Autodesk Inventor part; units mm, degrees
(part 2 of 4)
  line L125 (-9.1415, 0.6255) -> (-9.1721, 0.4922) construction
  line L126 (-9.1721, 0.4922) -> (-9.2026, 0.3592) construction
  line L127 (-9.2026, 0.3592) -> (-9.297, 0.2867) construction
  line L128 (-9.297, 0.2867) -> (-9.4268, 0.2624) construction
  line L129 (-9.4268, 0.2624) -> (-9.8787, 0.1776) construction
  line L130 (-9.8787, 0.1776) -> (-10.3313, 0.0968) construction
  line L131 (-10.3313, 0.0968) -> (-10.7828, 0.0101) construction
  line L132 (-10.7828, 0.0101) -> (-10.8726, -0.0072) construction
  line L133 (-10.8726, -0.0072) -> (-10.9599, -0.0407) construction
  line L134 (-10.9599, -0.0407) -> (-11.0464, -0.0719) construction
  line L135 (-11.0464, -0.0719) -> (-11.1372, -0.1048) construction
  line L136 (-11.1372, -0.1048) -> (-11.1793, -0.178) construction
  line L137 (-11.1793, -0.178) -> (-11.202, -0.269) construction
  line L138 (-11.202, -0.269) -> (-11.2438, -0.4368) construction
  line L139 (-11.2438, -0.4368) -> (-11.2023, -0.5985) construction
  line L140 (-11.2023, -0.5985) -> (-11.1712, -0.7605) construction
  line L141 (-11.1712, -0.7605) -> (-11.1015, -1.1234) construction
  line L142 (-11.1015, -1.1234) -> (-11.0295, -1.4858) construction
  line L143 (-11.0295, -1.4858) -> (-10.9532, -1.8473) construction
  line L144 (-10.9532, -1.8473) -> (-10.9457, -1.8828) construction
  line L145 (-10.9457, -1.8828) -> (-10.9084, -1.9273) construction
  line L146 (-10.9084, -1.9273) -> (-10.8748, -1.9396) construction
  line L147 (-10.8748, -1.9396) -> (-10.4566, -2.0916) construction
  line L148 (-10.4566, -2.0916) -> (-10.0419, -2.2568) construction
  line L149 (-10.0419, -2.2568) -> (-9.6157, -2.3822) construction
  line L150 (-9.6157, -2.3822) -> (-8.9721, -2.5716) construction
  line L151 (-8.9721, -2.5716) -> (-8.3199, -2.7319) construction
  line L152 (-8.3199, -2.7319) -> (-7.6717, -2.9059) construction
  line L153 (-7.6717, -2.9059) -> (-7.5951, -2.9264) construction
  line L154 (-7.5951, -2.9264) -> (-7.5555, -2.8808) construction
  line L155 (-7.5555, -2.8808) -> (-7.5235, -2.8285) construction
  line L156 (-7.5235, -2.8285) -> (-7.4397, -2.692) construction
  line L157 (-7.4397, -2.692) -> (-7.4153, -2.5388) construction
  line L158 (-7.4153, -2.5388) -> (-7.442, -2.3849) construction
  line L159 (-7.442, -2.3849) -> (-7.5081, -2.0041) construction
  line L160 (-7.5081, -2.0041) -> (-7.582, -1.6246) construction
  line L161 (-7.582, -1.6246) -> (-7.6571, -1.2454) construction
  line L162 (-7.6571, -1.2454) -> (-7.746, -0.7971) construction
  line L163 (-7.746, -0.7971) -> (-7.8402, -0.3498) construction
  line L164 (-7.8402, -0.3498) -> (-7.9309, 0.0982) construction
  line L165 (-7.9309, 0.0982) -> (-7.9807, 0.3436) construction
  line L166 (-7.9807, 0.3436) -> (-8.0916, 0.4464) construction
  line L167 (-8.0916, 0.4464) -> (-8.3387, 0.4678) construction
  line L168 (-8.3387, 0.4678) -> (-8.4163, 0.4745) construction
  line L169 (-8.4163, 0.4745) -> (-8.4944, 0.4741) construction
  line L170 (-8.4944, 0.4741) -> (-8.5722, 0.4792) construction
  line L171 (-8.5722, 0.4792) -> (-8.6303, 0.483) construction
  line L172 (-8.6303, 0.483) -> (-8.6898, 0.4839) construction
  line L173 (-8.6898, 0.4839) -> (-8.7459, 0.4976) construction
  line L174 (-8.7459, 0.4976) -> (-8.9235, 0.5409) construction
  line L175 (-8.9235, 0.5409) -> (-8.992, 0.7175) construction
  line L176 (-8.992, 0.7175) -> (-8.8985, 0.8745) construction
  line L177 (-8.8985, 0.8745) -> (-8.7942, 1.0494) construction
  line L178 (-8.7942, 1.0494) -> (-8.6225, 1.1165) construction
  line L179 (-8.6225, 1.1165) -> (-8.4386, 1.1526) construction
  line L180 (-8.4386, 1.1526) -> (-8.2405, 1.1914) construction
  line L181 (-8.2405, 1.1914) -> (-8.0393, 1.2145) construction
  line L182 (-8.0393, 1.2145) -> (-7.8391, 1.2422) construction
  line L183 (-7.8391, 1.2422) -> (-7.4652, 1.294) construction
  line L184 (-7.4652, 1.294) -> (-7.0916, 1.348) construction
  line L185 (-7.0916, 1.348) -> (-6.7169, 1.3925) construction
  line L186 (-6.7169, 1.3925) -> (-6.6023, 1.4061) construction
  line L187 (-6.6023, 1.4061) -> (-6.4832, 1.401) construction
  line L188 (-6.4832, 1.401) -> (-6.3682, 1.3875) construction
  line L189 (-6.3682, 1.3875) -> (-6.2267, 1.3709) construction
  line L190 (-6.2267, 1.3709) -> (-6.1216, 1.2721) construction
  line L191 (-6.1216, 1.2721) -> (-6.1023, 1.1616) construction
  line L192 (-6.1023, 1.1616) -> (-6.0806, 1.0381) construction
  line L193 (-6.0806, 1.0381) -> (-6.1476, 0.8994) construction
  line L194 (-6.1476, 0.8994) -> (-6.2789, 0.8383) construction
  line L195 (-6.2789, 0.8383) -> (-6.3816, 0.7906) construction
  line L196 (-6.3816, 0.7906) -> (-6.4934, 0.761) construction
  line L197 (-6.4934, 0.761) -> (-6.6033, 0.7308) construction
  line L198 (-6.6033, 0.7308) -> (-6.8238, 0.6701) construction
  line L199 (-6.8238, 0.6701) -> (-6.9226, 0.5484) construction
  line L200 (-6.9226, 0.5484) -> (-6.8975, 0.3204) construction
  line L201 (-6.8975, 0.3204) -> (-6.8633, 0.0086) construction
  line L202 (-6.8633, 0.0086) -> (-6.8208, -0.3026) construction
  line L203 (-6.8208, -0.3026) -> (-6.7684, -0.6118) construction
  line L204 (-6.7684, -0.6118) -> (-6.6783, -1.144) construction
  line L205 (-6.6783, -1.144) -> (-6.5786, -1.6746) construction
  line L206 (-6.5786, -1.6746) -> (-6.481, -2.2055) construction
  line L207 (-6.481, -2.2055) -> (-6.467, -2.2818) construction
  line L208 (-6.467, -2.2818) -> (-6.4462, -2.3575) construction
  line L209 (-6.4462, -2.3575) -> (-6.421, -2.4308) construction
  line L210 (-6.421, -2.4308) -> (-6.3423, -2.6595) construction
  line L211 (-6.3423, -2.6595) -> (-6.1706, -2.751) construction
  line L212 (-6.1706, -2.751) -> (-5.9336, -2.7011) construction
  line L213 (-5.9336, -2.7011) -> (-5.7911, -2.6711) construction
  line L214 (-5.7911, -2.6711) -> (-5.6477, -2.6422) construction
  line L215 (-5.6477, -2.6422) -> (-5.5032, -2.6256) construction
  line L216 (-5.5032, -2.6256) -> (-5.3654, -2.6098) construction
  line L217 (-5.3654, -2.6098) -> (-5.2355, -2.6427) construction
  line L218 (-5.2355, -2.6427) -> (-5.1342, -2.7463) construction
  line L219 (-5.1342, -2.7463) -> (-4.9562, -2.9286) construction
  line L220 (-4.9562, -2.9286) -> (-5.0397, -3.2467) construction
  line L221 (-5.0397, -3.2467) -> (-5.2961, -3.3506) construction
  line L222 (-5.2961, -3.3506) -> (-5.3877, -3.3877) construction
  line L223 (-5.3877, -3.3877) -> (-5.4863, -3.4076) construction
  line L224 (-5.4863, -3.4076) -> (-5.5964, -3.4396) construction
  line L225 (-5.5964, -3.4396) -> (-5.5666, -3.452) construction
  line L226 (-5.5666, -3.452) -> (-5.5456, -3.4636) construction
  line L227 (-5.5456, -3.4636) -> (-5.5231, -3.4696) construction
  line L228 (-5.5231, -3.4696) -> (-4.46, -3.7519) construction
  line L229 (-4.46, -3.7519) -> (-3.4059, -4.0644) construction
  line L230 (-3.4059, -4.0644) -> (-2.3654, -4.4212) construction
  line L231 (-2.3654, -4.4212) -> (-2.0639, -4.5246) construction
  line L232 (-2.0639, -4.5246) -> (-1.761, -4.6318) construction
  line L233 (-1.761, -4.6318) -> (-1.5003, -4.8214) construction
  line L234 (-1.5003, -4.8214) -> (-1.3917, -4.9004) construction
  line L235 (-1.3917, -4.9004) -> (-1.2877, -4.9957) construction
  line L236 (-1.2877, -4.9957) -> (-1.209, -5.1036) construction
  line L237 (-1.209, -5.1036) -> (-1.0533, -5.3173) construction
  line L238 (-1.0533, -5.3173) -> (-1.0838, -5.5776) construction
  line L239 (-1.0838, -5.5776) -> (-1.263, -5.7724) construction
  line L240 (-1.263, -5.7724) -> (-1.4413, -5.9664) construction
  line L241 (-1.4413, -5.9664) -> (-1.6684, -6.0667) construction
  line L242 (-1.6684, -6.0667) -> (-1.9231, -6.0989) construction
  line L243 (-1.9231, -6.0989) -> (-2.3941, -6.1586) construction
  line L244 (-2.3941, -6.1586) -> (-2.8652, -6.2281) construction
  line L245 (-2.8652, -6.2281) -> (-3.3385, -6.2567) construction
  line L246 (-3.3385, -6.2567) -> (-4.0167, -6.2976) construction
  line L247 (-4.0167, -6.2976) -> (-4.697, -6.3272) construction
  line L248 (-4.697, -6.3272) -> (-5.3762, -6.3227) construction
  line L249 (-5.3762, -6.3227) -> (-6.4798, -6.3154) construction
  line L250 (-6.4798, -6.3154) -> (-7.5831, -6.275) construction
  line L251 (-7.5831, -6.275) -> (-8.6866, -6.2514) construction
  line L252 (-8.6866, -6.2514) -> (-9.3078, -6.2382) construction
  line L253 (-9.3078, -6.2382) -> (-9.9297, -6.2097) construction
  line L254 (-9.9297, -6.2097) -> (-10.5503, -6.2255) construction
  line L255 (-10.5503, -6.2255) -> (-11.385, -6.2468) construction
  line L256 (-11.385, -6.2468) -> (-12.2071, -6.3678) construction
  line L257 (-12.2071, -6.3678) -> (-12.9983, -6.6549) construction
  line L258 (-12.9983, -6.6549) -> (-13.5047, -6.8387) construction
  line L259 (-13.5047, -6.8387) -> (-13.9638, -7.1106) construction
  line L260 (-13.9638, -7.1106) -> (-14.4209, -7.39) construction
  line L261 (-14.4209, -7.39) -> (-14.9749, -7.7284) construction
  line L262 (-14.9749, -7.7284) -> (-15.5263, -8.0734) construction
  line L263 (-15.5263, -8.0734) -> (-16.098, -8.38) construction
  line L264 (-16.098, -8.38) -> (-16.8167, -8.7655) construction
  line L265 (-16.8167, -8.7655) -> (-17.5898, -9.0139) construction
  line L266 (-17.5898, -9.0139) -> (-18.3874, -9.1846) construction
  line L267 (-18.3874, -9.1846) -> (-19.1584, -9.3496) construction
  line L268 (-19.1584, -9.3496) -> (-19.9377, -9.4137) construction
  line L269 (-19.9377, -9.4137) -> (-20.7253, -9.3901) construction
  line L270 (-20.7253, -9.3901) -> (-21.2696, -9.3737) construction
  line L271 (-21.2696, -9.3737) -> (-21.8068, -9.3051) construction
  line L272 (-21.8068, -9.3051) -> (-22.3409, -9.1993) construction
  line L273 (-22.3409, -9.1993) -> (-22.8994, -9.0886) construction
  line L274 (-22.8994, -9.0886) -> (-23.4408, -8.9244) construction
  line L275 (-23.4408, -8.9244) -> (-23.9614, -8.6965) construction
  line L276 (-23.9614, -8.6965) -> (-24.7827, -8.3369) construction
  line L277 (-24.7827, -8.3369) -> (-25.5451, -7.8792) construction
  line L278 (-25.5451, -7.8792) -> (-26.1979, -7.2599) construction
  line L279 (-26.1979, -7.2599) -> (-26.6165, -6.8628) construction
  line L280 (-26.6165, -6.8628) -> (-27.0112, -6.4405) construction
  line L281 (-27.0112, -6.4405) -> (-27.4171, -6.03) construction
  line L282 (-27.4171, -6.03) -> (-27.5073, -5.9388) construction
  line L283 (-27.5073, -5.9388) -> (-27.5995, -5.8496) construction
  line L284 (-27.5995, -5.8496) -> (-27.6907, -5.7595) construction
  line L285 (-27.6907, -5.7595) -> (-27.6972, -5.7631) construction
  line L286 (-27.6972, -5.7631) -> (-27.7038, -5.7666) construction
  line L287 (-27.7038, -5.7666) -> (-27.7103, -5.7702) construction
  line L288 (-27.7103, -5.7702) -> (-27.7045, -5.7909) construction
  line L289 (-27.7045, -5.7909) -> (-27.6981, -5.8114) construction
  line L290 (-27.6981, -5.8114) -> (-27.6931, -5.8323) construction
  line L291 (-27.6931, -5.8323) -> (-27.6517, -6.0067) construction
  line L292 (-27.6517, -6.0067) -> (-27.597, -6.1793) construction
  line L293 (-27.597, -6.1793) -> (-27.5727, -6.356) construction
  line L294 (-27.5727, -6.356) -> (-27.5432, -6.5712) construction
  line L295 (-27.5432, -6.5712) -> (-27.7159, -6.7223) construction
  line L296 (-27.7159, -6.7223) -> (-27.9327, -6.695) construction
  line L297 (-27.9327, -6.695) -> (-28.1066, -6.6731) construction
  line L298 (-28.1066, -6.6731) -> (-28.2563, -6.5942) construction
  line L299 (-28.2563, -6.5942) -> (-28.4029, -6.5055) construction
  line L300 (-28.4029, -6.5055) -> (-28.723, -6.312) construction
  line L301 (-28.723, -6.312) -> (-28.988, -6.0549) construction
  line L302 (-28.988, -6.0549) -> (-29.2411, -5.7836) construction
  line L303 (-29.2411, -5.7836) -> (-29.3886, -5.6255) construction
  line L304 (-29.3886, -5.6255) -> (-29.5283, -5.4582) construction
  line L305 (-29.5283, -5.4582) -> (-29.6891, -5.3148) construction
  line L306 (-29.6891, -5.3148) -> (-29.8892, -5.1361) construction
  line L307 (-29.8892, -5.1361) -> (-30.1284, -5.0394) construction
  line L308 (-30.1284, -5.0394) -> (-30.4054, -5.0607) construction
  line L309 (-30.4054, -5.0607) -> (-30.6564, -5.08) construction
  line L310 (-30.6564, -5.08) -> (-30.8625, -5.1824) construction
  line L311 (-30.8625, -5.1824) -> (-31.0209, -5.3798) construction
  line L312 (-31.0209, -5.3798) -> (-31.16, -5.5532) construction
  line L313 (-31.16, -5.5532) -> (-31.2551, -5.7489) construction
  line L314 (-31.2551, -5.7489) -> (-31.3218, -5.9595) construction
  line L315 (-31.3218, -5.9595) -> (-31.4388, -6.3288) construction
  line L316 (-31.4388, -6.3288) -> (-31.6164, -6.6694) construction
  line L317 (-31.6164, -6.6694) -> (-31.8243, -6.9939) construction
  line L318 (-31.8243, -6.9939) -> (-31.9164, -7.1375) construction
  line L319 (-31.9164, -7.1375) -> (-32.0288, -7.2696) construction
  line L320 (-32.0288, -7.2696) -> (-32.1781, -7.3575) construction
  line L321 (-32.1781, -7.3575) -> (-32.2423, -7.3953) construction
  line L322 (-32.2423, -7.3953) -> (-32.3224, -7.4185) construction
  line L323 (-32.3224, -7.4185) -> (-32.397, -7.4237) construction
  line L324 (-32.397, -7.4237) -> (-32.5113, -7.4317) construction
  line L325 (-32.5113, -7.4317) -> (-32.5926, -7.3729) construction
  line L326 (-32.5926, -7.3729) -> (-32.6412, -7.2633) construction
  line L327 (-32.6412, -7.2633) -> (-32.7533, -7.0109) construction
  line L328 (-32.7533, -7.0109) -> (-32.7522, -6.7457) construction
  line L329 (-32.7522, -6.7457) -> (-32.7292, -6.4807) construction
  line L330 (-32.7292, -6.4807) -> (-32.6561, -5.6383) construction
  line L331 (-32.6561, -5.6383) -> (-32.4383, -4.8295) construction
  line L332 (-32.4383, -4.8295) -> (-32.1464, -4.0389) construction
  line L333 (-32.1464, -4.0389) -> (-32.0867, -3.877) construction
  line L334 (-32.0867, -3.877) -> (-32.0244, -3.7159) construction
  line L335 (-32.0244, -3.7159) -> (-31.9579, -3.5566) construction
  line L336 (-31.9579, -3.5566) -> (-31.9347, -3.5009) construction
  line L337 (-31.9347, -3.5009) -> (-31.9455, -3.479) construction
  line L338 (-31.9455, -3.479) -> (-32.002, -3.4635) construction
  line L339 (-32.002, -3.4635) -> (-32.5597, -3.31) construction
  line L340 (-32.5597, -3.31) -> (-33.1132, -3.1393) construction
  line L341 (-33.1132, -3.1393) -> (-33.6753, -3.004) construction
  line L342 (-33.6753, -3.004) -> (-34.5429, -2.7951) construction
  line L343 (-34.5429, -2.7951) -> (-35.4166, -2.6112) construction
  line L344 (-35.4166, -2.6112) -> (-36.2872, -2.4147) construction
  line L345 (-36.2872, -2.4147) -> (-36.9812, -2.2582) construction
  line L346 (-36.9812, -2.2582) -> (-37.6646, -2.0653) construction
  line L347 (-37.6646, -2.0653) -> (-38.3233, -1.7938) construction
  line L348 (-38.3233, -1.7938) -> (-38.6564, -1.6565) construction
  line L349 (-38.6564, -1.6565) -> (-38.9816, -1.5016) construction
  line L350 (-38.9816, -1.5016) -> (-39.2782, -1.2935) construction
  line L351 (-39.2782, -1.2935) -> (-39.3873, -1.2169) construction
  line L352 (-39.3873, -1.2169) -> (-39.48, -1.1241) construction
  line L353 (-39.48, -1.1241) -> (-39.5354, -1.0006) construction
  line L354 (-39.5354, -1.0006) -> (-39.6222, -0.8072) construction
  line L355 (-39.6222, -0.8072) -> (-39.6072, -0.6192) construction
  line L356 (-39.6072, -0.6192) -> (-39.4623, -0.4639) construction
  line L357 (-39.4623, -0.4639) -> (-39.3816, -0.3774) construction
  line L358 (-39.3816, -0.3774) -> (-39.2771, -0.3041) construction
  line L359 (-39.2771, -0.3041) -> (-39.17, -0.2526) construction
  line L360 (-39.17, -0.2526) -> (-38.7966, -0.0731) construction
  line L361 (-38.7966, -0.0731) -> (-38.3904, -0.0146) construction
  line L362 (-38.3904, -0.0146) -> (-37.9851, 0.0411) construction
  line L363 (-37.9851, 0.0411) -> (-37.8502, 0.0596) construction
  line L364 (-37.8502, 0.0596) -> (-37.7138, 0.0677) construction
  line L365 (-37.7138, 0.0677) -> (-37.5779, 0.079) construction
  line L366 (-37.5779, 0.079) -> (-37.5311, 0.0828) construction
  line L367 (-37.5311, 0.0828) -> (-37.5181, 0.0974) construction
  line L368 (-37.5181, 0.0974) -> (-37.5278, 0.1486) construction
  line L369 (-37.5278, 0.1486) -> (-37.6076, 0.5737) construction
  line L370 (-37.6076, 0.5737) -> (-37.6983, 0.9976) construction
  line L371 (-37.6983, 0.9976) -> (-37.7568, 1.4258) construction
  line L372 (-37.7568, 1.4258) -> (-37.8162, 1.8607) construction
  line L373 (-37.8162, 1.8607) -> (-37.8234, 2.3001) construction
  line L374 (-37.8234, 2.3001) -> (-37.755, 2.737) construction
  line L375 (-37.755, 2.737) -> (-37.7344, 2.8688) construction
  line L376 (-37.7344, 2.8688) -> (-37.6587, 2.9608) construction
  line L377 (-37.6587, 2.9608) -> (-37.529, 2.9842) construction
  line L378 (-37.529, 2.9842) -> (-37.2061, 3.0425) construction
  line L379 (-37.2061, 3.0425) -> (-36.8828, 3.1064) construction
  line L380 (-36.8828, 3.1064) -> (-36.5568, 3.1378) construction
  line L381 (-36.5568, 3.1378) -> (-36.2765, 3.1648) construction
  line L382 (-36.2765, 3.1648) -> (-35.9921, 3.1533) construction
  line L383 (-35.9921, 3.1533) -> (-35.7096, 3.1523) construction
  line L384 (-35.7096, 3.1523) -> (-35.5311, 3.1516) construction
  line L385 (-35.5311, 3.1516) -> (-35.3544, 3.13) construction
  line L386 (-35.3544, 3.13) -> (-35.1948, 3.0392) construction
  line L387 (-35.1948, 3.0392) -> (-35.0805, 2.9741) construction
  line L388 (-35.0805, 2.9741) -> (-35.003, 2.8762) construction
  line L389 (-35.003, 2.8762) -> (-34.9516, 2.7566) construction
  line L390 (-34.9516, 2.7566) -> (-34.862, 2.5478) construction
  line L391 (-34.862, 2.5478) -> (-34.8252, 2.3278) construction
  line L392 (-34.8252, 2.3278) -> (-34.8157, 2.1027) construction
  line L393 (-34.8157, 2.1027) -> (-34.8121, 2.0169) construction
  line L394 (-34.8121, 2.0169) -> (-34.8151, 1.9308) construction
  line L395 (-34.8151, 1.9308) -> (-34.8151, 1.8449) construction
  line L396 (-34.8151, 1.8449) -> (-34.807, 1.8426) construction
  line L397 (-34.807, 1.8426) -> (-34.7989, 1.8403) construction
  line L398 (-34.7989, 1.8403) -> (-34.7908, 1.838) construction
  spline S1 degree 3 poles (-10.8046, -2.6746) (-10.8049, -2.6785) (-10.8072, -2.6879) (-10.8063, -2.6971) (-10.7803, -2.9734) (-10.75, -3.2493) (-10.7292, -3.526) (-10.7136, -3.7324) (-10.7319, -3.9357) (-10.8435, -4.1189) (-10.9866, -4.3539) (-11.2778, -4.4375) (-11.5015, -4.3033) (-11.6301, -4.2262) (-11.6996, -4.0978) (-11.7608, -3.9671) (-12.0323, -3.3866) (-12.1854, -2.772) (-12.271, -2.1401) (-12.2917, -1.9874) (-12.3401, -1.8815) (-12.4777, -1.7932) (-12.9915, -1.4638) (-13.4224, -1.0367) (-13.8361, -0.5922) (-13.8769, -0.5484) (-13.9189, -0.5326) (-13.9761, -0.5314) (-14.1048, -0.5288) (-14.2353, -0.5324) (-14.3617, -0.512) (-14.5586, -0.4803) (-14.6622, -0.2857) (-14.5841, -0.1023) (-14.5536, -0.0307) (-14.4987, 0.0306) (-14.4527, 0.0999) (-14.4997, 0.1558) (-14.5529, 0.2189) (-14.6061, 0.282) (-15.0566, 0.8164) (-15.5463, 1.3081) (-16.128, 1.7028) (-16.9784, 2.2798) (-17.9224, 2.6173) (-18.9269, 2.7951) (-19.2333, 2.8493) (-19.5445, 2.8822) (-19.8549, 2.906) (-20.3614, 2.9449) (-20.8673, 2.9238) (-21.3726, 2.8668) (-21.9816, 2.7981) (-22.5798, 2.6806) (-23.1623, 2.4911) (-23.7885, 2.2873) (-24.3706, 1.9875) (-24.9124, 1.618) (-25.3363, 1.3289) (-25.7398, 1.0097) (-26.1481, 0.6983) (-26.5739, 0.3736) (-27.0196, 0.0859) (-27.5287, -0.0923) (-28.2067, -0.3296) (-28.9059, -0.464) (-29.6225, -0.4881) (-30.1801, -0.5069) (-30.7387, -0.4944) (-31.2969, -0.499) (-31.3887, -0.4997) (-31.4802, -0.5174) (-31.5721, -0.5251) (-31.603, -0.5277) (-31.6347, -0.5254) (-31.6656, -0.5218) (-31.7232, -0.5152) (-31.7805, -0.4991) (-31.8379, -0.4988) (-32.5935, -0.4951) (-33.3492, -0.493) (-34.1048, -0.4917) (-34.4607, -0.4912) (-34.8166, -0.4966) (-35.1725, -0.4937) (-35.9986, -0.487) (-36.8248, -0.4755) (-37.6486, -0.5569) (-38.0343, -0.595) (-38.4189, -0.6404) (-38.7866, -0.773) (-38.8072, -0.7804) (-38.8243, -0.7973) (-38.8431, -0.8098) (-38.8262, -0.8253) (-38.8114, -0.8442) (-38.7922, -0.8558) (-38.4004, -1.092) (-37.9807, -1.2643) (-37.5477, -1.4089) (-36.9677, -1.6025) (-36.3767, -1.7518) (-35.7788, -1.8784) (-35.2435, -1.9918) (-34.7108, -2.1178) (-34.1767, -2.2372) (-33.3526, -2.4216) (-32.5354, -2.6318) (-31.7305, -2.8878) (-31.6684, -2.9076) (-31.6405, -2.8931) (-31.6079, -2.841) (-31.5371, -2.7276) (-31.4631, -2.6156) (-31.3819, -2.5095) (-31.2437, -2.3292) (-31.063, -2.2407) (-30.8323, -2.2878) (-30.6949, -2.3159) (-30.5688, -2.3726) (-30.4548, -2.4553) (-29.9506, -2.821) (-29.5224, -3.2668) (-29.1131, -3.7318) (-28.9127, -3.9595) (-28.7294, -4.1961) (-28.4587, -4.3589) (-28.1812, -4.5258) (-27.9327, -4.7411) (-27.6712, -4.9349) (-27.648, -4.9521) (-27.6226, -4.9665) (-27.5822, -4.9924) (-27.5822, -4.944) (-27.5788, -4.9155) (-27.5827, -4.888) (-27.6204, -4.6229) (-27.657, -4.3577) (-27.6982, -4.0931) (-27.7858, -3.5307) (-27.8782, -2.969) (-27.9632, -2.4061) (-27.9801, -2.2942) (-27.9893, -2.1758) (-27.9718, -2.0652) (-27.9482, -1.9157) (-27.8419, -1.823) (-27.6939, -1.7885) (-27.5471, -1.7543) (-27.4144, -1.7824) (-27.3043, -1.8935) (-27.1869, -2.012) (-27.1473, -2.1672) (-27.1107, -2.3201) (-27.0474, -2.5847) (-26.9969, -2.8525) (-26.9392, -3.1186) (-26.8342, -3.6032) (-26.7294, -4.0879) (-26.6212, -4.5718) (-26.5735, -4.7852) (-26.5279, -4.9999) (-26.4629, -5.2082) (-26.4002, -5.4087) (-26.2543, -5.5304) (-26.0386, -5.5436) (-25.9177, -5.551) (-25.7949, -5.5483) (-25.6742, -5.5369) (-25.2463, -5.4967) (-24.831, -5.3903) (-24.4153, -5.287) (-24.1563, -5.2226) (-23.8956, -5.1707) (-23.6286, -5.2246) (-23.3911, -5.2725) (-23.195, -5.3854) (-23.0898, -5.6166) (-23.0018, -5.8099) (-23.0739, -5.9575) (-23.2803, -6.0122) (-24.101, -6.2296) (-24.9399, -6.3475) (-25.7786, -6.4663) (-25.87, -6.4792) (-25.9618, -6.4898) (-26.067, -6.5032) (-26.0389, -6.5371) (-26.0252, -6.5571) (-26.0081, -6.5737) (-25.7001, -6.8723) (-25.376, -7.1519) (-25.0219, -7.3949) (-24.3485, -7.8571) (-23.6204, -8.2039) (-22.8349, -8.4301) (-22.3167, -8.5793) (-21.79, -8.6915) (-21.2532, -8.7308) (-20.8485, -8.7604) (-20.44, -8.7586) (-20.034, -8.7452) (-19.4221, -8.7251) (-18.8161, -8.6439) (-18.22, -8.4998) (-17.4595, -8.3159) (-16.7344, -8.0394) (-16.0583, -7.6444) (-15.5733, -7.361) (-15.0953, -7.0654) (-14.6164, -6.7717) (-14.1471, -6.484) (-13.6663, -6.2202) (-13.1436, -6.0411) (-12.3452, -5.7674) (-11.5228, -5.6253) (-10.6798, -5.6092) (-9.8536, -5.5933) (-9.0279, -5.6198) (-8.2018, -5.6397) (-7.0916, -5.6664) (-5.982, -5.7441) (-4.8705, -5.7013) (-4.4493, -5.6851) (-4.0273, -5.6778) (-3.6074, -5.6442) (-3.0858, -5.6025) (-2.5658, -5.5397) (-2.0456, -5.4809) (-1.9626, -5.4714) (-1.8825, -5.4349) (-1.8011, -5.4109) (-1.8021, -5.4025) (-1.8031, -5.3941) (-1.8041, -5.3857) (-1.823, -5.3711) (-1.8401, -5.3529) (-1.861, -5.3426) (-2.0349, -5.2564) (-2.2024, -5.1502) (-2.385, -5.0902) (-3.152, -4.8384) (-3.9203, -4.5897) (-4.6943, -4.3607) (-5.3937, -4.1537) (-6.1028, -3.9797) (-6.8041, -3.7791) (-7.0583, -3.7064) (-7.3037, -3.6819) (-7.5647, -3.7375) (-7.7779, -3.7828) (-7.9978, -3.8063) (-8.2158, -3.8169) (-8.473, -3.8294) (-8.6584, -3.5989) (-8.5873, -3.3635) (-8.5839, -3.3524) (-8.5838, -3.3404) (-8.5835, -3.3387) (-9.3253, -3.1169) (-10.0622, -2.8966) (-10.8046, -2.6746) knots 0 0 0 0 1 1 1 2 2 2 3 3 3 4 4 4 5 5 5 6 6 6 7 7 7 8 8 8 9 9 9 10 10 10 11 11 11 12 12 12 13 13 13 14 14 14 15 15 15 16 16 16 17 17 17 18 18 18 19 19 19 20 20 20 21 21 21 22 22 22 23 23 23 24 24 24 25 25 25 26 26 26 27 27 27 28 28 28 29 29 29 30 30 30 31 31 31 32 32 32 33 33 33 34 34 34 35 35 35 36 36 36 37 37 37 38 38 38 39 39 39 40 40 40 41 41 41 42 42 42 43 43 43 44 44 44 45 45 45 46 46 46 47 47 47 48 48 48 49 49 49 50 50 50 51 51 51 52 52 52 53 53 53 54 54 54 55 55 55 56 56 56 57 57 57 58 58 58 59 59 59 60 60 60 61 61 61 62 62 62 63 63 63 64 64 64 65 65 65 66 66 66 67 67 67 68 68 68 69 69 69 70 70 70 71 71 71 72 72 72 73 73 73 74 74 74 75 75 75 76 76 76 77 77 77 78 78 78 79 79 79 80 80 80 81 81 81 82 82 82 83 83 83 84 84 84 85 85 85 86 86 86 87 87 87 87
  line L399 (-10.8046, -2.6746) -> (-10.8049, -2.6785) construction
  line L400 (-10.8049, -2.6785) -> (-10.8072, -2.6879) construction
  line L401 (-10.8072, -2.6879) -> (-10.8063, -2.6971) construction
  line L402 (-10.8063, -2.6971) -> (-10.7803, -2.9734) construction
  line L403 (-10.7803, -2.9734) -> (-10.75, -3.2493) construction
  line L404 (-10.75, -3.2493) -> (-10.7292, -3.526) construction
  line L405 (-10.7292, -3.526) -> (-10.7136, -3.7324) construction
  line L406 (-10.7136, -3.7324) -> (-10.7319, -3.9357) construction
  line L407 (-10.7319, -3.9357) -> (-10.8435, -4.1189) construction
  line L408 (-10.8435, -4.1189) -> (-10.9866, -4.3539) construction
  line L409 (-10.9866, -4.3539) -> (-11.2778, -4.4375) construction
  line L410 (-11.2778, -4.4375) -> (-11.5015, -4.3033) construction
  line L411 (-11.5015, -4.3033) -> (-11.6301, -4.2262) construction
  line L412 (-11.6301, -4.2262) -> (-11.6996, -4.0978) construction
  line L413 (-11.6996, -4.0978) -> (-11.7608, -3.9671) construction
  line L414 (-11.7608, -3.9671) -> (-12.0323, -3.3866) construction
  line L415 (-12.0323, -3.3866) -> (-12.1854, -2.772) construction
  line L416 (-12.1854, -2.772) -> (-12.271, -2.1401) construction
  line L417 (-12.271, -2.1401) -> (-12.2917, -1.9874) construction
  line L418 (-12.2917, -1.9874) -> (-12.3401, -1.8815) construction
  line L419 (-12.3401, -1.8815) -> (-12.4777, -1.7932) construction
  line L420 (-12.4777, -1.7932) -> (-12.9915, -1.4638) construction
  line L421 (-12.9915, -1.4638) -> (-13.4224, -1.0367) construction
  line L422 (-13.4224, -1.0367) -> (-13.8361, -0.5922) construction
  line L423 (-13.8361, -0.5922) -> (-13.8769, -0.5484) construction
  line L424 (-13.8769, -0.5484) -> (-13.9189, -0.5326) construction
  line L425 (-13.9189, -0.5326) -> (-13.9761, -0.5314) construction
  line L426 (-13.9761, -0.5314) -> (-14.1048, -0.5288) construction
  line L427 (-14.1048, -0.5288) -> (-14.2353, -0.5324) construction
  line L428 (-14.2353, -0.5324) -> (-14.3617, -0.512) construction
  line L429 (-14.3617, -0.512) -> (-14.5586, -0.4803) construction
  line L430 (-14.5586, -0.4803) -> (-14.6622, -0.2857) construction
  line L431 (-14.6622, -0.2857) -> (-14.5841, -0.1023) construction
  line L432 (-14.5841, -0.1023) -> (-14.5536, -0.0307) construction
  line L433 (-14.5536, -0.0307) -> (-14.4987, 0.0306) construction
  line L434 (-14.4987, 0.0306) -> (-14.4527, 0.0999) construction
  line L435 (-14.4527, 0.0999) -> (-14.4997, 0.1558) construction
  line L436 (-14.4997, 0.1558) -> (-14.5529, 0.2189) construction
  line L437 (-14.5529, 0.2189) -> (-14.6061, 0.282) construction
  line L438 (-14.6061, 0.282) -> (-15.0566, 0.8164) construction
  line L439 (-15.0566, 0.8164) -> (-15.5463, 1.3081) construction
  line L440 (-15.5463, 1.3081) -> (-16.128, 1.7028) construction
  line L441 (-16.128, 1.7028) -> (-16.9784, 2.2798) construction
  line L442 (-16.9784, 2.2798) -> (-17.9224, 2.6173) construction
  line L443 (-17.9224, 2.6173) -> (-18.9269, 2.7951) construction
  line L444 (-18.9269, 2.7951) -> (-19.2333, 2.8493) construction
  line L445 (-19.2333, 2.8493) -> (-19.5445, 2.8822) construction
  line L446 (-19.5445, 2.8822) -> (-19.8549, 2.906) construction
  line L447 (-19.8549, 2.906) -> (-20.3614, 2.9449) construction
  line L448 (-20.3614, 2.9449) -> (-20.8673, 2.9238) construction
  line L449 (-20.8673, 2.9238) -> (-21.3726, 2.8668) construction
  line L450 (-21.3726, 2.8668) -> (-21.9816, 2.7981) construction
  line L451 (-21.9816, 2.7981) -> (-22.5798, 2.6806) construction
  line L452 (-22.5798, 2.6806) -> (-23.1623, 2.4911) construction
  line L453 (-23.1623, 2.4911) -> (-23.7885, 2.2873) construction
  line L454 (-23.7885, 2.2873) -> (-24.3706, 1.9875) construction
  line L455 (-24.3706, 1.9875) -> (-24.9124, 1.618) construction
  line L456 (-24.9124, 1.618) -> (-25.3363, 1.3289) construction
  line L457 (-25.3363, 1.3289) -> (-25.7398, 1.0097) construction
  line L458 (-25.7398, 1.0097) -> (-26.1481, 0.6983) construction
  line L459 (-26.1481, 0.6983) -> (-26.5739, 0.3736) construction
  line L460 (-26.5739, 0.3736) -> (-27.0196, 0.0859) construction
  line L461 (-27.0196, 0.0859) -> (-27.5287, -0.0923) construction
  line L462 (-27.5287, -0.0923) -> (-28.2067, -0.3296) construction
  line L463 (-28.2067, -0.3296) -> (-28.9059, -0.464) construction
  line L464 (-28.9059, -0.464) -> (-29.6225, -0.4881) construction
  line L465 (-29.6225, -0.4881) -> (-30.1801, -0.5069) construction
  line L466 (-30.1801, -0.5069) -> (-30.7387, -0.4944) construction
  line L467 (-30.7387, -0.4944) -> (-31.2969, -0.499) construction
  line L468 (-31.2969, -0.499) -> (-31.3887, -0.4997) construction
  line L469 (-31.3887, -0.4997) -> (-31.4802, -0.5174) construction
  line L470 (-31.4802, -0.5174) -> (-31.5721, -0.5251) construction
  line L471 (-31.5721, -0.5251) -> (-31.603, -0.5277) construction
  line L472 (-31.603, -0.5277) -> (-31.6347, -0.5254) construction
  line L473 (-31.6347, -0.5254) -> (-31.6656, -0.5218) construction
  line L474 (-31.6656, -0.5218) -> (-31.7232, -0.5152) construction
  line L475 (-31.7232, -0.5152) -> (-31.7805, -0.4991) construction
  line L476 (-31.7805, -0.4991) -> (-31.8379, -0.4988) construction
  line L477 (-31.8379, -0.4988) -> (-32.5935, -0.4951) construction
  line L478 (-32.5935, -0.4951) -> (-33.3492, -0.493) construction
  line L479 (-33.3492, -0.493) -> (-34.1048, -0.4917) construction
  line L480 (-34.1048, -0.4917) -> (-34.4607, -0.4912) construction
  line L481 (-34.4607, -0.4912) -> (-34.8166, -0.4966) construction
  line L482 (-34.8166, -0.4966) -> (-35.1725, -0.4937) construction
  line L483 (-35.1725, -0.4937) -> (-35.9986, -0.487) construction
  line L484 (-35.9986, -0.487) -> (-36.8248, -0.4755) construction
  line L485 (-36.8248, -0.4755) -> (-37.6486, -0.5569) construction
  line L486 (-37.6486, -0.5569) -> (-38.0343, -0.595) construction
  line L487 (-38.0343, -0.595) -> (-38.4189, -0.6404) construction
  line L488 (-38.4189, -0.6404) -> (-38.7866, -0.773) construction
  line L489 (-38.7866, -0.773) -> (-38.8072, -0.7804) construction
  line L490 (-38.8072, -0.7804) -> (-38.8243, -0.7973) construction
  line L491 (-38.8243, -0.7973) -> (-38.8431, -0.8098) construction
  line L492 (-38.8431, -0.8098) -> (-38.8262, -0.8253) construction
  line L493 (-38.8262, -0.8253) -> (-38.8114, -0.8442) construction
  line L494 (-38.8114, -0.8442) -> (-38.7922, -0.8558) construction
  line L495 (-38.7922, -0.8558) -> (-38.4004, -1.092) construction
  line L496 (-38.4004, -1.092) -> (-37.9807, -1.2643) construction
  line L497 (-37.9807, -1.2643) -> (-37.5477, -1.4089) construction
  line L498 (-37.5477, -1.4089) -> (-36.9677, -1.6025) construction
  line L499 (-36.9677, -1.6025) -> (-36.3767, -1.7518) construction
  line L500 (-36.3767, -1.7518) -> (-35.7788, -1.8784) construction
  line L501 (-35.7788, -1.8784) -> (-35.2435, -1.9918) construction
  line L502 (-35.2435, -1.9918) -> (-34.7108, -2.1178) construction
  line L503 (-34.7108, -2.1178) -> (-34.1767, -2.2372) construction
  line L504 (-34.1767, -2.2372) -> (-33.3526, -2.4216) construction
  line L505 (-33.3526, -2.4216) -> (-32.5354, -2.6318) construction
  line L506 (-32.5354, -2.6318) -> (-31.7305, -2.8878) construction
  line L507 (-31.7305, -2.8878) -> (-31.6684, -2.9076) construction
  line L508 (-31.6684, -2.9076) -> (-31.6405, -2.8931) construction
  line L509 (-31.6405, -2.8931) -> (-31.6079, -2.841) construction
  line L510 (-31.6079, -2.841) -> (-31.5371, -2.7276) construction
  line L511 (-31.5371, -2.7276) -> (-31.4631, -2.6156) construction
  line L512 (-31.4631, -2.6156) -> (-31.3819, -2.5095) construction
  line L513 (-31.3819, -2.5095) -> (-31.2437, -2.3292) construction
  line L514 (-31.2437, -2.3292) -> (-31.063, -2.2407) construction
  line L515 (-31.063, -2.2407) -> (-30.8323, -2.2878) construction
  line L516 (-30.8323, -2.2878) -> (-30.6949, -2.3159) construction
  line L517 (-30.6949, -2.3159) -> (-30.5688, -2.3726) construction
  line L518 (-30.5688, -2.3726) -> (-30.4548, -2.4553) construction
  line L519 (-30.4548, -2.4553) -> (-29.9506, -2.821) construction
  line L520 (-29.9506, -2.821) -> (-29.5224, -3.2668) construction
  line L521 (-29.5224, -3.2668) -> (-29.1131, -3.7318) construction
  line L522 (-29.1131, -3.7318) -> (-28.9127, -3.9595) construction
  line L523 (-28.9127, -3.9595) -> (-28.7294, -4.1961) construction
  line L524 (-28.7294, -4.1961) -> (-28.4587, -4.3589) construction
  line L525 (-28.4587, -4.3589) -> (-28.1812, -4.5258) construction
  line L526 (-28.1812, -4.5258) -> (-27.9327, -4.7411) construction
  line L527 (-27.9327, -4.7411) -> (-27.6712, -4.9349) construction
  line L528 (-27.6712, -4.9349) -> (-27.648, -4.9521) construction
  line L529 (-27.648, -4.9521) -> (-27.6226, -4.9665) construction
  line L530 (-27.6226, -4.9665) -> (-27.5822, -4.9924) construction
  line L531 (-27.5822, -4.9924) -> (-27.5822, -4.944) construction
  line L532 (-27.5822, -4.944) -> (-27.5788, -4.9155) construction
  line L533 (-27.5788, -4.9155) -> (-27.5827, -4.888) construction
  line L534 (-27.5827, -4.888) -> (-27.6204, -4.6229) construction
  line L535 (-27.6204, -4.6229) -> (-27.657, -4.3577) construction
  line L536 (-27.657, -4.3577) -> (-27.6982, -4.0931) construction
  line L537 (-27.6982, -4.0931) -> (-27.7858, -3.5307) construction
  line L538 (-27.7858, -3.5307) -> (-27.8782, -2.969) construction
  line L539 (-27.8782, -2.969) -> (-27.9632, -2.4061) construction
  line L540 (-27.9632, -2.4061) -> (-27.9801, -2.2942) construction
  line L541 (-27.9801, -2.2942) -> (-27.9893, -2.1758) construction
  line L542 (-27.9893, -2.1758) -> (-27.9718, -2.0652) construction
  line L543 (-27.9718, -2.0652) -> (-27.9482, -1.9157) construction
  line L544 (-27.9482, -1.9157) -> (-27.8419, -1.823) construction
  line L545 (-27.8419, -1.823) -> (-27.6939, -1.7885) construction
  line L546 (-27.6939, -1.7885) -> (-27.5471, -1.7543) construction
  line L547 (-27.5471, -1.7543) -> (-27.4144, -1.7824) construction
  line L548 (-27.4144, -1.7824) -> (-27.3043, -1.8935) construction
  line L549 (-27.3043, -1.8935) -> (-27.1869, -2.012) construction
  line L550 (-27.1869, -2.012) -> (-27.1473, -2.1672) construction
  line L551 (-27.1473, -2.1672) -> (-27.1107, -2.3201) construction
  line L552 (-27.1107, -2.3201) -> (-27.0474, -2.5847) construction
  line L553 (-27.0474, -2.5847) -> (-26.9969, -2.8525) construction
  line L554 (-26.9969, -2.8525) -> (-26.9392, -3.1186) construction
  line L555 (-26.9392, -3.1186) -> (-26.8342, -3.6032) construction
  line L556 (-26.8342, -3.6032) -> (-26.7294, -4.0879) construction
  line L557 (-26.7294, -4.0879) -> (-26.6212, -4.5718) construction
  line L558 (-26.6212, -4.5718) -> (-26.5735, -4.7852) construction
  line L559 (-26.5735, -4.7852) -> (-26.5279, -4.9999) construction
  line L560 (-26.5279, -4.9999) -> (-26.4629, -5.2082) construction
  line L561 (-26.4629, -5.2082) -> (-26.4002, -5.4087) construction
  line L562 (-26.4002, -5.4087) -> (-26.2543, -5.5304) construction
  line L563 (-26.2543, -5.5304) -> (-26.0386, -5.5436) construction
  line L564 (-26.0386, -5.5436) -> (-25.9177, -5.551) construction
  line L565 (-25.9177, -5.551) -> (-25.7949, -5.5483) construction
  line L566 (-25.7949, -5.5483) -> (-25.6742, -5.5369) construction
  line L567 (-25.6742, -5.5369) -> (-25.2463, -5.4967) construction
  line L568 (-25.2463, -5.4967) -> (-24.831, -5.3903) construction
  line L569 (-24.831, -5.3903) -> (-24.4153, -5.287) construction
  line L570 (-24.4153, -5.287) -> (-24.1563, -5.2226) construction
  line L571 (-24.1563, -5.2226) -> (-23.8956, -5.1707) construction
  line L572 (-23.8956, -5.1707) -> (-23.6286, -5.2246) construction
  line L573 (-23.6286, -5.2246) -> (-23.3911, -5.2725) construction
  line L574 (-23.3911, -5.2725) -> (-23.195, -5.3854) construction
  line L575 (-23.195, -5.3854) -> (-23.0898, -5.6166) construction
  line L576 (-23.0898, -5.6166) -> (-23.0018, -5.8099) construction
  line L577 (-23.0018, -5.8099) -> (-23.0739, -5.9575) construction
  line L578 (-23.0739, -5.9575) -> (-23.2803, -6.0122) construction
  line L579 (-23.2803, -6.0122) -> (-24.101, -6.2296) construction
  line L580 (-24.101, -6.2296) -> (-24.9399, -6.3475) construction
  line L581 (-24.9399, -6.3475) -> (-25.7786, -6.4663) construction
  line L582 (-25.7786, -6.4663) -> (-25.87, -6.4792) construction
  line L583 (-25.87, -6.4792) -> (-25.9618, -6.4898) construction
  line L584 (-25.9618, -6.4898) -> (-26.067, -6.5032) construction
  line L585 (-26.067, -6.5032) -> (-26.0389, -6.5371) construction
  line L586 (-26.0389, -6.5371) -> (-26.0252, -6.5571) construction
  line L587 (-26.0252, -6.5571) -> (-26.0081, -6.5737) construction
  line L588 (-26.0081, -6.5737) -> (-25.7001, -6.8723) construction
  line L589 (-25.7001, -6.8723) -> (-25.376, -7.1519) construction
  line L590 (-25.376, -7.1519) -> (-25.0219, -7.3949) construction
  line L591 (-25.0219, -7.3949) -> (-24.3485, -7.8571) construction
  line L592 (-24.3485, -7.8571) -> (-23.6204, -8.2039) construction
  line L593 (-23.6204, -8.2039) -> (-22.8349, -8.4301) construction
  line L594 (-22.8349, -8.4301) -> (-22.3167, -8.5793) construction
  line L595 (-22.3167, -8.5793) -> (-21.79, -8.6915) construction
  line L596 (-21.79, -8.6915) -> (-21.2532, -8.7308) construction
  line L597 (-21.2532, -8.7308) -> (-20.8485, -8.7604) construction
  line L598 (-20.8485, -8.7604) -> (-20.44, -8.7586) construction
  line L599 (-20.44, -8.7586) -> (-20.034, -8.7452) construction
  line L600 (-20.034, -8.7452) -> (-19.4221, -8.7251) construction
  line L601 (-19.4221, -8.7251) -> (-18.8161, -8.6439) construction
  line L602 (-18.8161, -8.6439) -> (-18.22, -8.4998) construction
  line L603 (-18.22, -8.4998) -> (-17.4595, -8.3159) construction
  line L604 (-17.4595, -8.3159) -> (-16.7344, -8.0394) construction
  line L605 (-16.7344, -8.0394) -> (-16.0583, -7.6444) construction
  line L606 (-16.0583, -7.6444) -> (-15.5733, -7.361) construction
  line L607 (-15.5733, -7.361) -> (-15.0953, -7.0654) construction
  line L608 (-15.0953, -7.0654) -> (-14.6164, -6.7717) construction
  line L609 (-14.6164, -6.7717) -> (-14.1471, -6.484) construction
  line L610 (-14.1471, -6.484) -> (-13.6663, -6.2202) construction
  line L611 (-13.6663, -6.2202) -> (-13.1436, -6.0411) construction
  line L612 (-13.1436, -6.0411) -> (-12.3452, -5.7674) construction
  line L613 (-12.3452, -5.7674) -> (-11.5228, -5.6253) construction
  line L614 (-11.5228, -5.6253) -> (-10.6798, -5.6092) construction
  line L615 (-10.6798, -5.6092) -> (-9.8536, -5.5933) construction
  line L616 (-9.8536, -5.5933) -> (-9.0279, -5.6198) construction
  line L617 (-9.0279, -5.6198) -> (-8.2018, -5.6397) construction
  line L618 (-8.2018, -5.6397) -> (-7.0916, -5.6664) construction
  line L619 (-7.0916, -5.6664) -> (-5.982, -5.7441) construction
  line L620 (-5.982, -5.7441) -> (-4.8705, -5.7013) construction
  line L621 (-4.8705, -5.7013) -> (-4.4493, -5.6851) construction
  line L622 (-4.4493, -5.6851) -> (-4.0273, -5.6778) construction
  line L623 (-4.0273, -5.6778) -> (-3.6074, -5.6442) construction
  line L624 (-3.6074, -5.6442) -> (-3.0858, -5.6025) construction
  line L625 (-3.0858, -5.6025) -> (-2.5658, -5.5397) construction
  line L626 (-2.5658, -5.5397) -> (-2.0456, -5.4809) construction
  line L627 (-2.0456, -5.4809) -> (-1.9626, -5.4714) construction
  line L628 (-1.9626, -5.4714) -> (-1.8825, -5.4349) construction
  line L629 (-1.8825, -5.4349) -> (-1.8011, -5.4109) construction
  line L630 (-1.8011, -5.4109) -> (-1.8021, -5.4025) construction
  line L631 (-1.8021, -5.4025) -> (-1.8031, -5.3941) construction
  line L632 (-1.8031, -5.3941) -> (-1.8041, -5.3857) construction
  line L633 (-1.8041, -5.3857) -> (-1.823, -5.3711) construction
  line L634 (-1.823, -5.3711) -> (-1.8401, -5.3529) construction
  line L635 (-1.8401, -5.3529) -> (-1.861, -5.3426) construction
  line L636 (-1.861, -5.3426) -> (-2.0349, -5.2564) construction
  line L637 (-2.0349, -5.2564) -> (-2.2024, -5.1502) construction
  line L638 (-2.2024, -5.1502) -> (-2.385, -5.0902) construction
  line L639 (-2.385, -5.0902) -> (-3.152, -4.8384) construction
  line L640 (-3.152, -4.8384) -> (-3.9203, -4.5897) construction
  line L641 (-3.9203, -4.5897) -> (-4.6943, -4.3607) construction
  line L642 (-4.6943, -4.3607) -> (-5.3937, -4.1537) construction
  line L643 (-5.3937, -4.1537) -> (-6.1028, -3.9797) construction
  line L644 (-6.1028, -3.9797) -> (-6.8041, -3.7791) construction
  line L645 (-6.8041, -3.7791) -> (-7.0583, -3.7064) construction
  line L646 (-7.0583, -3.7064) -> (-7.3037, -3.6819) construction
  line L647 (-7.3037, -3.6819) -> (-7.5647, -3.7375) construction
  line L648 (-7.5647, -3.7375) -> (-7.7779, -3.7828) construction
  line L649 (-7.7779, -3.7828) -> (-7.9978, -3.8063) construction
  line L650 (-7.9978, -3.8063) -> (-8.2158, -3.8169) construction
  line L651 (-8.2158, -3.8169) -> (-8.473, -3.8294) construction
  line L652 (-8.473, -3.8294) -> (-8.6584, -3.5989) construction
  line L653 (-8.6584, -3.5989) -> (-8.5873, -3.3635) construction
  line L654 (-8.5873, -3.3635) -> (-8.5839, -3.3524) construction
  line L655 (-8.5839, -3.3524) -> (-8.5838, -3.3404) construction
  line L656 (-8.5838, -3.3404) -> (-8.5835, -3.3387) construction
  line L657 (-8.5835, -3.3387) -> (-9.3253, -3.1169) construction
  line L658 (-9.3253, -3.1169) -> (-10.0622, -2.8966) construction
  line L659 (-10.0622, -2.8966) -> (-10.8046, -2.6746) construction
  spline S2 degree 3 poles (-36.9183, 1.2424) (-36.9146, 1.2037) (-36.91, 1.1614) (-36.9065, 1.1191) (-36.8811, 0.8134) (-36.855, 0.5079) (-36.8315, 0.2021) (-36.8273, 0.1474) (-36.8096, 0.1264) (-36.7512, 0.1286) (-36.5712, 0.1357) (-36.3909, 0.139) (-36.2107, 0.1399) (-35.9136, 0.1414) (-35.6164, 0.138) (-35.3193, 0.1406) (-35.1758, 0.1419) (-35.1823, 0.1473) (-35.1557, 0.2864) (-35.0965, 0.5966) (-35.0299, 0.9055) (-34.9669, 1.215) (-34.9615, 1.2412) (-34.9598, 1.2682) (-34.9579, 1.283) (-35.0599, 1.235) (-35.1542, 1.1676) (-35.2581, 1.146) (-35.57, 1.0809) (-35.8877, 1.079) (-36.203, 1.1193) (-36.4382, 1.1494) (-36.6709, 1.199) (-36.9183, 1.2424) knots 0 0 0 0 1 1 1 2 2 2 3 3 3 4 4 4 5 5 5 6 6 6 7 7 7 8 8 8 9 9 9 10 10 10 11 11 11 11
  line L660 (-36.9183, 1.2424) -> (-36.9146, 1.2037) construction
  line L661 (-36.9146, 1.2037) -> (-36.91, 1.1614) construction
  line L662 (-36.91, 1.1614) -> (-36.9065, 1.1191) construction
  line L663 (-36.9065, 1.1191) -> (-36.8811, 0.8134) construction
  line L664 (-36.8811, 0.8134) -> (-36.855, 0.5079) construction
  line L665 (-36.855, 0.5079) -> (-36.8315, 0.2021) construction
  line L666 (-36.8315, 0.2021) -> (-36.8273, 0.1474) construction
  line L667 (-36.8273, 0.1474) -> (-36.8096, 0.1264) construction
  line L668 (-36.8096, 0.1264) -> (-36.7512, 0.1286) construction
  line L669 (-36.7512, 0.1286) -> (-36.5712, 0.1357) construction
  line L670 (-36.5712, 0.1357) -> (-36.3909, 0.139) construction
  line L671 (-36.3909, 0.139) -> (-36.2107, 0.1399) construction
  line L672 (-36.2107, 0.1399) -> (-35.9136, 0.1414) construction
  line L673 (-35.9136, 0.1414) -> (-35.6164, 0.138) construction
  line L674 (-35.6164, 0.138) -> (-35.3193, 0.1406) construction
  line L675 (-35.3193, 0.1406) -> (-35.1758, 0.1419) construction
  line L676 (-35.1758, 0.1419) -> (-35.1823, 0.1473) construction
  line L677 (-35.1823, 0.1473) -> (-35.1557, 0.2864) construction
  line L678 (-35.1557, 0.2864) -> (-35.0965, 0.5966) construction
  line L679 (-35.0965, 0.5966) -> (-35.0299, 0.9055) construction
  line L680 (-35.0299, 0.9055) -> (-34.9669, 1.215) construction
  line L681 (-34.9669, 1.215) -> (-34.9615, 1.2412) construction
  line L682 (-34.9615, 1.2412) -> (-34.9598, 1.2682) construction
  line L683 (-34.9598, 1.2682) -> (-34.9579, 1.283) construction
  line L684 (-34.9579, 1.283) -> (-35.0599, 1.235) construction
  line L685 (-35.0599, 1.235) -> (-35.1542, 1.1676) construction
  line L686 (-35.1542, 1.1676) -> (-35.2581, 1.146) construction
  line L687 (-35.2581, 1.146) -> (-35.57, 1.0809) construction
  line L688 (-35.57, 1.0809) -> (-35.8877, 1.079) construction
  line L689 (-35.8877, 1.079) -> (-36.203, 1.1193) construction
  line L690 (-36.203, 1.1193) -> (-36.4382, 1.1494) construction
  line L691 (-36.4382, 1.1494) -> (-36.6709, 1.199) construction
  line L692 (-36.6709, 1.199) -> (-36.9183, 1.2424) construction
  spline S3 degree 3 poles (-30.21, 0.1155) (-30.2276, 0.1466) (-30.235, 0.1635) (-30.2457, 0.1781) (-30.4571, 0.4669) (-30.6662, 0.7573) (-30.8818, 1.0429) (-30.9887, 1.1846) (-31.105, 1.3198) (-31.2641, 1.4089) (-31.3153, 1.4376) (-31.3526, 1.4281) (-31.3602, 1.3699) (-31.3737, 1.2669) (-31.3905, 1.1624) (-31.386, 1.0594) (-31.3731, 0.7652) (-31.3492, 0.4716) (-31.3324, 0.1776) (-31.3296, 0.129) (-31.3106, 0.1141) (-31.2655, 0.1151) (-31.1802, 0.1169) (-31.0949, 0.1155) (-31.0096, 0.1155) (-30.749, 0.1155) (-30.4884, 0.1155) (-30.21, 0.1155) knots 0 0 0 0 1 1 1 2 2 2 3 3 3 4 4 4 5 5 5 6 6 6 7 7 7 8 8 8 9 9 9 9
  line L693 (-30.21, 0.1155) -> (-30.2276, 0.1466) construction
  line L694 (-30.2276, 0.1466) -> (-30.235, 0.1635) construction
  line L695 (-30.235, 0.1635) -> (-30.2457, 0.1781) construction
  line L696 (-30.2457, 0.1781) -> (-30.4571, 0.4669) construction
  line L697 (-30.4571, 0.4669) -> (-30.6662, 0.7573) construction
  line L698 (-30.6662, 0.7573) -> (-30.8818, 1.0429) construction
  line L699 (-30.8818, 1.0429) -> (-30.9887, 1.1846) construction
  line L700 (-30.9887, 1.1846) -> (-31.105, 1.3198) construction
  line L701 (-31.105, 1.3198) -> (-31.2641, 1.4089) construction
  line L702 (-31.2641, 1.4089) -> (-31.3153, 1.4376) construction
  line L703 (-31.3153, 1.4376) -> (-31.3526, 1.4281) construction
  line L704 (-31.3526, 1.4281) -> (-31.3602, 1.3699) construction
  line L705 (-31.3602, 1.3699) -> (-31.3737, 1.2669) construction
  line L706 (-31.3737, 1.2669) -> (-31.3905, 1.1624) construction
  line L707 (-31.3905, 1.1624) -> (-31.386, 1.0594) construction
  line L708 (-31.386, 1.0594) -> (-31.3731, 0.7652) construction
  line L709 (-31.3731, 0.7652) -> (-31.3492, 0.4716) construction
  line L710 (-31.3492, 0.4716) -> (-31.3324, 0.1776) construction
  line L711 (-31.3324, 0.1776) -> (-31.3296, 0.129) construction
  line L712 (-31.3296, 0.129) -> (-31.3106, 0.1141) construction
  line L713 (-31.3106, 0.1141) -> (-31.2655, 0.1151) construction
  line L714 (-31.2655, 0.1151) -> (-31.1802, 0.1169) construction
  line L715 (-31.1802, 0.1169) -> (-31.0949, 0.1155) construction
  line L716 (-31.0949, 0.1155) -> (-31.0096, 0.1155) construction
  line L717 (-31.0096, 0.1155) -> (-30.749, 0.1155) construction
  line L718 (-30.749, 0.1155) -> (-30.4884, 0.1155) construction
  line L719 (-30.4884, 0.1155) -> (-30.21, 0.1155) construction
  spline S4 degree 3 poles (-33.0561, 0.1374) (-33.0687, 0.1623) (-33.0787, 0.1836) (-33.0901, 0.2041) (-33.155, 0.3209) (-33.2162, 0.4401) (-33.2866, 0.5536) (-33.3543, 0.6625) (-33.4206, 0.7759) (-33.5072, 0.8689) (-33.6943, 1.0697) (-33.9271, 1.0395) (-34.0848, 0.8154) (-34.1924, 0.6625) (-34.2271, 0.4812) (-34.3009, 0.3155) (-34.3243, 0.2629) (-34.3433, 0.2083) (-34.3711, 0.1374) (-33.9277, 0.1374) (-33.4981, 0.1374) (-33.0561, 0.1374) knots 0 0 0 0 1 1 1 2 2 2 3 3 3 4 4 4 5 5 5 6 6 6 7 7 7 7
  line L720 (-33.0561, 0.1374) -> (-33.0687, 0.1623) construction
  line L721 (-33.0687, 0.1623) -> (-33.0787, 0.1836) construction
  line L722 (-33.0787, 0.1836) -> (-33.0901, 0.2041) construction
  line L723 (-33.0901, 0.2041) -> (-33.155, 0.3209) construction
  line L724 (-33.155, 0.3209) -> (-33.2162, 0.4401) construction
  line L725 (-33.2162, 0.4401) -> (-33.2866, 0.5536) construction
  line L726 (-33.2866, 0.5536) -> (-33.3543, 0.6625) construction
  line L727 (-33.3543, 0.6625) -> (-33.4206, 0.7759) construction
  line L728 (-33.4206, 0.7759) -> (-33.5072, 0.8689) construction
  line L729 (-33.5072, 0.8689) -> (-33.6943, 1.0697) construction
  line L730 (-33.6943, 1.0697) -> (-33.9271, 1.0395) construction
  line L731 (-33.9271, 1.0395) -> (-34.0848, 0.8154) construction
  line L732 (-34.0848, 0.8154) -> (-34.1924, 0.6625) construction
  line L733 (-34.1924, 0.6625) -> (-34.2271, 0.4812) construction
  line L734 (-34.2271, 0.4812) -> (-34.3009, 0.3155) construction
  line L735 (-34.3009, 0.3155) -> (-34.3243, 0.2629) construction
  line L736 (-34.3243, 0.2629) -> (-34.3433, 0.2083) construction
  line L737 (-34.3433, 0.2083) -> (-34.3711, 0.1374) construction
  line L738 (-34.3711, 0.1374) -> (-33.9277, 0.1374) construction
  line L739 (-33.9277, 0.1374) -> (-33.4981, 0.1374) construction
  line L740 (-33.4981, 0.1374) -> (-33.0561, 0.1374) construction
  spline S5 degree 3 poles (-36.3665, 2.404) (-36.5139, 2.3856) (-36.6449, 2.3755) (-36.7734, 2.3514) (-36.8786, 2.3317) (-36.9052, 2.2737) (-36.8694, 2.1765) (-36.8552, 2.1379) (-36.8358, 2.1011) (-36.8212, 2.0626) (-36.7965, 1.9968) (-36.752, 1.9602) (-36.6802, 1.9558) (-36.5155, 1.9456) (-36.351, 1.9258) (-36.1863, 1.9252) (-36.0465, 1.9246) (-35.9064, 1.9438) (-35.767, 1.9589) (-35.7495, 1.9609) (-35.7233, 1.9899) (-35.7209, 2.009) (-35.7008, 2.1678) (-35.7931, 2.3069) (-35.9501, 2.3398) (-36.0921, 2.3695) (-36.2371, 2.3846) (-36.3665, 2.404) knots 0 0 0 0 1 1 1 2 2 2 3 3 3 4 4 4 5 5 5 6 6 6 7 7 7 8 8 8 9 9 9 9
  line L741 (-36.3665, 2.404) -> (-36.5139, 2.3856) construction
  line L742 (-36.5139, 2.3856) -> (-36.6449, 2.3755) construction
  line L743 (-36.6449, 2.3755) -> (-36.7734, 2.3514) construction
  line L744 (-36.7734, 2.3514) -> (-36.8786, 2.3317) construction
  line L745 (-36.8786, 2.3317) -> (-36.9052, 2.2737) construction
  line L746 (-36.9052, 2.2737) -> (-36.8694, 2.1765) construction
  line L747 (-36.8694, 2.1765) -> (-36.8552, 2.1379) construction
  line L748 (-36.8552, 2.1379) -> (-36.8358, 2.1011) construction